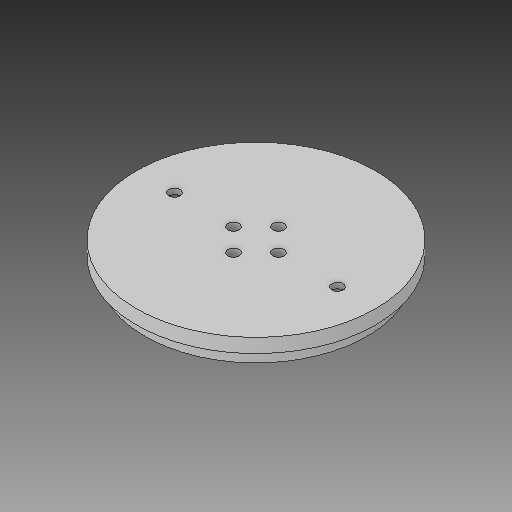
# Autodesk Inventor part: joint2_rotate_mec_patr2
Saved by Autodesk Inventor 2019 (Build 230136000, 136)
## iProperties
Created: 2019-12-26
Part Number: joint2_rotate_mec_patr2
Material: Типовые
Document SubType Name: Modeling
Designer: Петров Иван
Density: 1 g/cm^3
Appearance: По умолчанию
Author: Петров Иван
Autodesk Inventor part; units mm, degrees
ref_plane "YZ Plane" through (0, 0, 0) normal (1, 0, 0) x (0, 1, 0)
ref_plane "XZ Plane" through (0, 0, 0) normal (0, 1, 0) x (-1, 0, 0)
ref_plane "XY Plane" through (0, 0, 0) normal (0, 0, 1) x (1, 0, 0)
sketch "Эскиз1" plane through (0, 0, 0) normal (0, 1, 0) x (-1, 0, 0)
  circle A0 centre (0, 0) radius 39.5
  circle A1 centre (0, 0) radius 35.5
  dimension "d0" = 79
  dimension "d1" = 71
  constraints: 2 centre point, 2 coincident
  measures "d0" diameter of A0
  measures "d1" diameter of A1
extrude "Выдавливание1" add sketch "Эскиз1" along normal blind 5
sketch "Эскиз2" plane through (0, 5, 0) normal (0, 1, 0) x (1, 0, 0)
  circle A0 centre (0, 0) radius 42.5
  dimension "d4" = 85
  constraints: 1 centre point, 1 coincident
  measures "d4" diameter of A0
extrude "Выдавливание2" add sketch "Эскиз2" along normal blind 5
sketch "Эскиз3" plane through (0, 10, 0) normal (0, 1, 0) x (1, 0, 0)
  line L0 (0, 0) -> (-8, 0)
  circle A0 centre (-8, 0) radius 2
  dimension "d7" = 8
  dimension "d8" = 4
  constraints: 2 end point, 1 centre point, 1 coincident, 1 horizontal
  measures "d7" distance of L0.start L0.end
  measures "d8" diameter of A0
extrude "Выдавливание3" cut sketch "Эскиз3" against normal blind 5
pattern_circular "Круговой массив1" count 4 over 360 about axis through (0, 5, 0) along (0, 1, 0) of "Выдавливание3"
sketch "Эскиз4" plane through (0, 10, 0) normal (0, 1, 0) x (1, 0, 0)
  line L0 (0, 0) -> (-29, 0)
  circle A0 centre (-29, 0) radius 2
  line L1 (0, 0) -> (0, 42.5)
  circle A1 centre (0, 0) radius 42.5 projected
  dimension "d14" = 29
  dimension "d15" = 4
  dimension "d21" = 90
  constraints: 4 end point, 2 vertical, 1 centre point, 1 coincident, 1 vertical alignment, 1 other
  measures "d14" distance of point (0, 0) L0.end
  measures "d15" diameter of A0
  measures "d21" angle of L0 L1
extrude "Выдавливание4" cut sketch "Эскиз4" against normal blind 10 contours A0
pattern_circular "Круговой массив3" count 2 over 360 about axis through (0, 5, 0) along (0, 1, 0) of "Выдавливание4"
sketch "Эскиз5" plane through (0, 5, 0) normal (0, -1, 0) x (1, 0, 0)
  circle A0 centre (29, 0) radius 2 projected
  circle A1 centre (29, 0) radius 6.5
  circle A2 centre (-29, 0) radius 2 projected
  circle A3 centre (-29, 0) radius 6.5
  point P0 (0, 0)
  constraints: 2 centre point, 2 coincident
extrude "Выдавливание5" cut sketch "Эскиз5" against normal blind 3
sketch "Эскиз6" plane through (0, 10, 0) normal (0, 1, 0) x (1, 0, 0)
  circle A0 centre (29, 0) radius 2 projected
  circle A1 centre (-29, 0) radius 2 projected
  circle A2 centre (0, 8) radius 2 projected
  circle A3 centre (8, 0) radius 2 projected
  circle A4 centre (0, -8) radius 2 projected
  circle A5 centre (-8, 0) radius 2 projected
  circle A6 centre (0, 0) radius 42.5 projected
